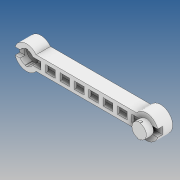
# Autodesk Inventor part: 1stopien
Saved by Autodesk Inventor 2022.3 (Build 263350000, 350)
## iProperties
Created: 2023-06-25
Part Number: 1stopien
Material: Tworzywo sztuczne ABS
Document SubType Name: Modeling
Designer: Chyba Ja
Density: 1.06 g/cm^3
Appearance: Gładki — biały
Author: Chyba Ja
Autodesk Inventor part; units mm, degrees
ref_plane "YZ Plane" through (0, 0, 0) normal (1, 0, 0) x (0, 1, 0)
ref_plane "XZ Plane" through (0, 0, 0) normal (0, 1, 0) x (-1, 0, 0)
ref_plane "XY Plane" through (0, 0, 0) normal (0, 0, 1) x (1, 0, 0)
sketch "Szkic1" plane through (0, 0, 0) normal (0, 0, 1) x (1, 0, 0)
  arc A0 (20, 15) -> (-20, 15) centre (0, 0) ccw
  line L0 (20, 15) -> (125, 15)
  line L1 (125, 15) -> (125, -15)
  line L2 (125, -15) -> (20, -15)
  arc A1 (230, -15) -> (230, 15) centre (250, 0) ccw
  line L3 (230, 15) -> (125, 15)
  line L4 (125, -15) -> (230, -15)
  arc A2 (-20, 15) -> (20, -15) centre (0, 0) ccw
  dimension "d0" = 50
  dimension "d1" = 30
  dimension "d2" = 250
  constraints: 10 end point, 6 point on circle, 5 symmetric about line, 4 coincident, 3 centre point, 1 horizontal, 1 parallel, 1 perpendicular, 1 point on line, 1 vertical alignment, 1 other
  measures "d0" diameter of A0
  measures "d1" distance between parallel lines of L2 L0
  measures "d2" distance of point (0, 0) point (250, 0)
extrude "kształt" add sketch "Szkic1" along normal blind 30
sketch "Szkic2" plane through (0, 0, 30) normal (0, 0, 1) x (1, 0, 0)
  arc A0 (20, 15) -> (20, -15) centre (0, 0) ccw projected
  line L0 (20, -15) -> (230, -15) projected
  arc A1 (230, -15) -> (230, 15) centre (250, 0) ccw projected
  line L1 (230, 15) -> (20, 15) projected
  line L2 (-23.8485, 7.5) -> (273.8485, 7.5)
  line L3 (273.8485, -7.5) -> (-23.8485, -7.5)
  point P0 (-23.8485, -7.5)
  dimension "d5" = 15
  constraints: 4 end point, 3 point on circle, 1 horizontal, 1 parallel, 1 vertical alignment
  measures "d5" distance between parallel lines of L3 L2
extrude "rowek na kable" cut sketch "Szkic2" against normal blind 10 contours L2 A1 L3 A0
sketch "Szkic3" plane through (0, 0, 30) normal (0, 0, 1) x (1, 0, 0)
  arc A0 (273.8485, 7.5) -> (230, 15) centre (250, 0) ccw projected
  circle A1 centre (250, 0) radius 15
  point P0 (0, 0)
  dimension "d8" = 30
  constraints: 1 centre point, 1 coincident
  measures "d8" diameter of A1
extrude "odstająćy cosik" add sketch "Szkic3" along normal blind 15
sketch "Szkic4" plane through (0, 0, 30) normal (0, 0, 1) x (1, 0, 0)
  circle A0 centre (0, 0) radius 15
  dimension "d11" = 30
  constraints: 1 centre point, 1 coincident
  measures "d11" diameter of A0
extrude "wgłebiający cosik" cut sketch "Szkic4" against normal blind 15
sketch "Szkic5" plane through (0, 0, 30) normal (0, 0, 1) x (1, 0, 0)
  arc A0 (12.9904, 7.5) -> (-12.9904, 7.5) centre (0, 0) ccw projected
  line L0 (12.9904, 7.5) -> (237.0096, 7.5) projected
  arc A1 (262.9904, 7.5) -> (237.0096, 7.5) centre (250, 0) ccw projected
  line L1 (262.9904, 7.5) -> (273.8485, 7.5) projected
  arc A2 (273.8485, 7.5) -> (230, 15) centre (250, 0) ccw projected
  line L2 (230, 15) -> (20, 15) projected
  arc A3 (20, 15) -> (-23.8485, 7.5) centre (0, 0) ccw projected
  line L3 (-23.8485, 7.5) -> (-12.9904, 7.5) projected
  arc A4 (-12.9904, -7.5) -> (12.9904, -7.5) centre (0, 0) ccw projected
  line L4 (-12.9904, -7.5) -> (-23.8485, -7.5) projected
  arc A5 (-23.8485, -7.5) -> (20, -15) centre (0, 0) ccw projected
  line L5 (20, -15) -> (230, -15) projected
  arc A6 (230, -15) -> (273.8485, -7.5) centre (250, 0) ccw projected
  line L6 (273.8485, -7.5) -> (262.9904, -7.5) projected
  arc A7 (237.0096, -7.5) -> (262.9904, -7.5) centre (250, 0) ccw projected
  line L7 (237.0096, -7.5) -> (12.9904, -7.5) projected
  line L8 (30, 7.5) -> (40, 7.5)
  line L9 (40, 7.5) -> (40, -7.5)
  line L10 (40, -7.5) -> (30, -7.5)
  line L11 (30, -7.5) -> (30, 7.5)
  arc A8 (-23.8485, -7.5) -> (20, -15) centre (0, 0) ccw projected
  line L12 (60, -7.5) -> (60, 7.5)
  line L13 (70, 7.5) -> (70, -7.5)
  line L14 (70, -7.5) -> (60, -7.5)
  line L15 (60, 7.5) -> (70, 7.5)
  line L16 (90, -7.5) -> (90, 7.5)
  line L17 (100, 7.5) -> (100, -7.5)
  line L18 (100, -7.5) -> (90, -7.5)
  line L19 (90, 7.5) -> (100, 7.5)
  line L20 (120, -7.5) -> (120, 7.5)
  line L21 (130, 7.5) -> (130, -7.5)
  line L22 (130, -7.5) -> (120, -7.5)
  line L23 (120, 7.5) -> (130, 7.5)
  line L24 (150, -7.5) -> (150, 7.5)
  line L25 (160, 7.5) -> (160, -7.5)
  line L26 (160, -7.5) -> (150, -7.5)
  line L27 (150, 7.5) -> (160, 7.5)
  line L28 (180, -7.5) -> (180, 7.5)
  line L29 (190, 7.5) -> (190, -7.5)
  line L30 (190, -7.5) -> (180, -7.5)
  line L31 (180, 7.5) -> (190, 7.5)
  line L32 (210, -7.5) -> (210, 7.5)
  line L33 (220, 7.5) -> (220, -7.5)
  line L34 (220, -7.5) -> (210, -7.5)
  line L35 (210, 7.5) -> (220, 7.5)
  arc A9 (273.8485, 7.5) -> (230, 15) centre (250, 0) ccw projected
  line L36 (0, 0) -> (125, 0) construction
  line L37 (125, -7.5) -> (125, 7.5) construction
  line L38 (125, 0) -> (250, 0) construction
  point P0 (70, -7.5)
  point P1 (60, 7.5)
  point P2 (220, -7.5)
  point P3 (210, 7.5)
  point P4 (190, -7.5)
  point P5 (180, 7.5)
  point P6 (160, -7.5)
  point P7 (150, 7.5)
  point P8 (130, -7.5)
  point P9 (120, 7.5)
  point P10 (100, -7.5)
  point P11 (90, 7.5)
  dimension "d15" = 10
  dimension "d18" = 30
  constraints: 62 end point, 4 horizontal, 3 midpoint, 2 parallel, 2 perpendicular, 2 point on line, 1 collinear, 49 other
  measures "d15" distance between parallel lines of L11 L9
  measures "d18" distance of L10.end L12.start
extrude "wzmocnienie" add sketch "Szkic5" against normal blind 5 contours L0 L9 L7 L11 | L0 L13 L7 L12 | L0 L17 L7 L16 | L0 L21 L7 L20 | L33 L7 L32 L0 | L0 L25 L7 L24 | L29 L7 L28 L0
sketch "Szkic6" plane through (250, 0, 45) normal (0, 0, 1) x (1, 0, 0)
  circle A0 centre (0, 0) radius 15 projected
  arc A1 (2.5, 15.8035) -> (2.5, -15.8035) centre (0, 0) ccw construction
  line L0 (-2.5, 15.8035) -> (2.5, 15.8035)
  line L1 (2.5, 15.8035) -> (2.5, 14.7902)
  line L2 (2.5, -15.8035) -> (-2.5, -15.8035)
  line L3 (-2.5, -15.8035) -> (-2.5, -14.7902)
  line L4 (2.5, 14.7902) -> (2.5, -14.7902) construction
  line L5 (-2.5, 14.7902) -> (-2.5, 15.8035)
  line L6 (-2.5, -14.7902) -> (-2.5, 14.7902) construction
  line L7 (2.5, -14.7902) -> (2.5, -15.8035)
  point P0 (-250, 0)
  dimension "d25" = 32
  dimension "d27" = 5
  constraints: 16 end point, 10 parallel, 8 point on circle, 3 perpendicular, 2 horizontal alignment, 1 centre point, 1 coincident, 1 horizontal
  measures "d25" diameter of A1
  measures "d27" distance between parallel lines of L6 L4
extrude "Wyciągnięcie proste6" add sketch "Szkic6" against normal blind 5 contours A0 L5 L0 L1 | L7 L2 L3 A0
sketch "Szkic7" plane through (0, 0, 30) normal (0, 0, 1) x (1, 0, 0)
  circle A0 centre (0, 0) radius 16 construction
  line L0 (-2.5, 15.8035) -> (2.5, 15.8035)
  line L1 (2.5, -15.8035) -> (-2.5, -15.8035)
  arc A1 (12.9904, 7.5) -> (-12.9904, 7.5) centre (0, 0) ccw projected
  arc A2 (-12.9904, -7.5) -> (12.9904, -7.5) centre (0, 0) ccw projected
  line L2 (2.5, 15.8035) -> (2.5, 14.7902)
  line L3 (2.5, -14.7902) -> (2.5, -15.8035)
  line L4 (-2.5, -15.8035) -> (-2.5, -14.7902)
  line L5 (-2.5, 14.7902) -> (-2.5, 15.8035)
  arc A3 (2.5, 14.7902) -> (-2.5, 14.7902) centre (0, 0) ccw
  arc A4 (-2.5, -14.7902) -> (2.5, -14.7902) centre (0, 0) ccw
  point P0 (2.5, 15.2968)
  dimension "d30" = 32
  dimension "d32" = 5
  constraints: 12 end point, 11 point on circle, 5 parallel, 3 centre point, 2 coincident, 2 collinear, 2 perpendicular, 1 horizontal, 1 midpoint
  measures "d30" diameter of A0
  measures "d32" distance from line of L5 point (2.5, 15.297)
extrude "Wyciągnięcie proste7" cut sketch "Szkic7" against normal up to surface (15 mm away)
